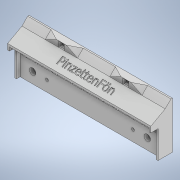
# Autodesk Inventor part: Leitung3-b
Saved by Autodesk Inventor 2020 (Build 240168000, 168)
## iProperties
Created: 2019-09-12
Part Number: Leitung3-b
Material: Generic
Document SubType Name: Modeling
Designer: rainer
Density: 1 g/cm^3
Appearance: Default
Author: rainer
Autodesk Inventor part; units mm, degrees
ref_plane "YZ Plane" through (0, 0, 0) normal (1, 0, 0) x (0, 1, 0)
ref_plane "XZ Plane" through (0, 0, 0) normal (0, 1, 0) x (-1, 0, 0)
sketch "Sketch1" plane through (0, 0, 0) normal (0, 0, 1) x (1, 0, 0)
  line L0 (-100, 17.5) -> (100, 17.5)
  line L1 (100, 17.5) -> (100, -17.5)
  line L2 (100, -17.5) -> (-100, -17.5)
  line L3 (-100, -17.5) -> (-100, 17.5)
  point P0 (0, 0)
  point P1 (0, 17.5)
  point P2 (-100, 0)
  dimension "d0" = 200
  dimension "d1" = 35
  constraints: 8 end point, 2 midpoint, 2 parallel, 1 horizontal, 1 horizontal alignment, 1 perpendicular, 1 vertical alignment
  measures "d0" distance of L0.start L0.end
  measures "d1" distance of L2.end L0.start
extrude "Extrusion1" add sketch "Sketch1" along normal blind 10
ref_plane "Work Plane1" through (0, 0, 30) normal (0, 0, 1) x (1, 0, 0)
sketch "Sketch2" plane through (0, 0, 30) normal (0, 0, 1) x (1, 0, 0)
  line L0 (-100, -17.5) -> (100, -17.5)
  line L1 (100, -17.5) -> (100, 6.5)
  line L2 (100, 6.5) -> (-100, 6.5)
  line L3 (-100, 6.5) -> (-100, -17.5)
  line L4 (100, 17.5) -> (-100, 17.5) projected
  line L5 (-100, -17.5) -> (100, -17.5) projected
  point P0 (0, 0)
  point P1 (0, 6.5)
  dimension "d5" = 24
  dimension "d6" = 200
  dimension "d32" = 0
  constraints: 8 end point, 2 parallel, 1 horizontal, 1 midpoint, 1 perpendicular, 1 vertical alignment
  measures "d5" distance of L2.end L0.start
  measures "d6" distance of L1.end L2.end
  measures "d32" distance between parallel lines of L5 L0
extrude "Extrusion2" add sketch "Sketch2" along normal blind 10
loft "Loft1" add section 1 edges at (0, -17.5, 10) (100, 0, 10) (0, 17.5, 10) (-100, 0, 10) section 2 edges at (0, -17.5, 30) (-100, -5.5, 30) (0, 6.5, 30) (100, -5.5, 30)
sketch "Sketch3" plane through (0, 0, 0) normal (0, 0, -1) x (-1, 0, 0)
  line L0 (-95, 12.5) -> (95, 12.5)
  line L1 (95, 12.5) -> (95, -12.5)
  line L2 (95, -12.5) -> (-95, -12.5)
  line L3 (-95, -12.5) -> (-95, 12.5)
  point P0 (0, 0)
  point P1 (-95, 0)
  point P2 (0, 12.5)
  dimension "d14" = 190
  dimension "d15" = 25
  constraints: 8 end point, 2 midpoint, 2 parallel, 1 horizontal, 1 horizontal alignment, 1 perpendicular, 1 vertical alignment
  measures "d14" distance of L0.start L0.end
  measures "d15" distance of L2.end L0.start
extrude "Extrusion3" cut sketch "Sketch3" against normal blind 10
sketch "Sketch4" plane through (0, 0, 40) normal (0, 0, 1) x (1, 0, 0)
  line L0 (-95, -12.5) -> (95, -12.5)
  line L1 (95, -12.5) -> (95, 3.5)
  line L2 (95, 3.5) -> (-95, 3.5)
  line L3 (-95, 3.5) -> (-95, -12.5)
  line L4 (-100, -17.5) -> (100, -17.5) projected
  point P0 (0, 0)
  point P1 (0, 3.5)
  dimension "d18" = 190
  dimension "d19" = 16
  dimension "d20" = 5
  constraints: 8 end point, 2 parallel, 1 horizontal, 1 midpoint, 1 perpendicular, 1 vertical alignment
  measures "d18" distance of L1.end L2.end
  measures "d19" distance of L2.end L0.start
  measures "d20" distance between parallel lines of L4 L0
extrude "Extrusion4" cut sketch "Sketch4" against normal blind 10
loft "Loft3" cut section 1 edges at (0, 3.5, 30) (-95, -4.5, 30) (0, -12.5, 30) (95, -4.5, 30) section 2 edges at (-95, 0, 10) (0, 12.5, 10) (95, 0, 10) (0, -12.5, 10)
sketch "Sketch6" plane through (0, 0, 40) normal (0, 0, 1) x (1, 0, 0)
  line L0 (-109.7574, -25.248) -> (108.0798, -25.248)
  line L1 (108.0798, -25.248) -> (108.0798, 3.5)
  line L2 (108.0798, 3.5) -> (-109.7574, 3.5)
  line L3 (-109.7574, 3.5) -> (-109.7574, -25.248)
  point P0 (0, 0)
  constraints: 8 end point, 2 parallel, 1 horizontal, 1 perpendicular
extrude "Extrusion6" cut sketch "Sketch6" against normal blind 25
thicken "Thicken2" operation add thickness 10 both sides no extend neighbours yes toward (0, 0, -1) faces at (33.3333, 4.5, 40)
sketch "Sketch7" plane through (-100, -17.5, 0) normal (0, -1, 0) x (1, 0, 0)
  line L0 (200, 0) -> (0, 0) projected
  line L1 (200, 15) -> (0, 15) projected
  line L2 (10, 0) -> (50, 0)
  line L3 (50, 0) -> (50, 15)
  line L4 (50, 15) -> (10, 15)
  line L5 (10, 15) -> (10, 0)
  line L6 (0, 0) -> (0, 15) projected
  line L7 (190, 0) -> (150, 0)
  line L8 (150, 0) -> (150, 15)
  line L9 (150, 15) -> (190, 15)
  line L10 (190, 15) -> (190, 0)
  line L11 (200, 0) -> (200, 15) projected
  point P0 (100, 0)
  point P1 (190, 15)
  point P2 (150, 0)
  point P3 (10, 15)
  dimension "d41" = 40
  dimension "d42" = 10
  dimension "d43" = 40
  dimension "d44" = 10
  constraints: 16 end point, 4 parallel, 4 point on line, 2 horizontal, 2 perpendicular
  measures "d41" distance between parallel lines of L3 L5
  measures "d42" distance between parallel lines of L6 L5
  measures "d43" distance between parallel lines of L10 L8
  measures "d44" distance between parallel lines of L11 L10
extrude "Extrusion7" add sketch "Sketch7" along normal blind 15 contours L0 L8 L1 L10 | L0 L5 L1 L3
sketch "Sketch9" plane through (0, 0, 15) normal (0, 0, 1) x (1, 0, 0)
  line L0 (-90, -17.5) -> (-90, -32.5) projected
  line L1 (-50, -32.5) -> (-90, -32.5) projected
  line L2 (90, -32.5) -> (50, -32.5) projected
  line L3 (50, -17.5) -> (50, -32.5) projected
  line L4 (90, -17.5) -> (90, -32.5) projected
  point P0 (0, 0)
  point P1 (-80, -25)
  point P2 (80, -25)
  dimension "d62" = 10
  dimension "d63" = 7.5
  dimension "d64" = 7.5
  dimension "d73" = 10
  measures "d62" distance from line of L0 point (-80, -25)
  measures "d63" distance from line of L1 point (-80, -25)
  measures "d64" distance from line of L2 point (80, -25)
  measures "d73" distance from line of L4 point (80, -25)
hole "Hole2" at (-80, -25, 15) at (80, -25, 15) direction (0, 0, -1) diameter 4.2 end through all counterbore diameter 9 counterbore depth 5
sketch "Sketch10" plane through (0, 0, 15) normal (0, 0, 1) x (1, 0, 0)
  line L0 (-50, -17.5) -> (-50, -32.5) projected
  line L1 (-50, -32.5) -> (-90, -32.5) projected
  line L2 (50, -17.5) -> (50, -32.5) projected
  point P0 (0, 0)
  point P1 (-60, -25)
  point P2 (60, -25)
  dimension "d74" = 10
  dimension "d75" = 7.5
  dimension "d76" = 10
  measures "d74" distance from line of L0 point (-60, -25)
  measures "d75" distance from line of L1 point (-60, -25)
  measures "d76" distance from line of L2 point (60, -25)
hole "Hole3" at (-60, -25, 15) at (60, -25, 15) direction (0, 0, -1) diameter 4.2 end through all
sketch "Sketch11" plane through (0, 0, 0) normal (0, 0, -1) x (-1, 0, 0)
  line L0 (95, -12.5) -> (-95, -12.5) projected
  line L1 (-95, 12.5) -> (95, 12.5) projected
  line L2 (-75.6667, -12.5) -> (-73.6667, -12.5)
  line L3 (-73.6667, -12.5) -> (-73.6667, 12.5)
  line L4 (-73.6667, 12.5) -> (-75.6667, 12.5)
  line L5 (-75.6667, 12.5) -> (-75.6667, -12.5)
  line L6 (-95, -12.5) -> (-95, 12.5) projected
  point P0 (0, 0)
  dimension "d84" = 2
  dimension "d85" = 19.3333
  constraints: 8 end point, 2 parallel, 2 point on line, 1 horizontal, 1 perpendicular
  measures "d84" distance between parallel lines of L3 L5
  measures "d85" distance between parallel lines of L6 L5
extrude "Extrusion8" add sketch "Sketch11" against normal blind 30 contours L0 L5 L1 L3
pattern_linear "Rectangular Pattern1" count 8 spacing 21.3333 along (-1, 0, 0) of "Extrusion8"
sketch "Sketch12" plane through (100, -17.5, 0) normal (1, 0, 0) x (0, 0, -1)
  line L0 (-30, 21) -> (-30, 24) projected
  line L1 (0, 35) -> (-10, 35) projected
  line L2 (-30, 24) -> (-10, 35)
  line L3 (-10, 35) -> (-34.2959, 35)
  line L4 (-34.2959, 35) -> (-33.7888, 23.828)
  line L5 (-33.7888, 23.828) -> (-30, 24)
  point P0 (0, 17.5)
  constraints: 8 end point, 1 collinear, 1 perpendicular
extrude "Extrusion9" cut sketch "Sketch12" against normal through all
sketch "Sketch13" plane through (100, -17.5, 0) normal (1, 0, 0) x (0, 0, -1)
  line L0 (-31.9216, 3.0257) -> (-15, 3.0257)
  line L1 (-15, 3.0257) -> (-15, 20)
  line L2 (-15, 20) -> (-31.9216, 20)
  line L3 (-31.9216, 20) -> (-31.9216, 3.0257)
  line L4 (-30, 21) -> (-15, 21) projected
  line L5 (-15, 21) -> (-15, 0) projected
  point P0 (0, 17.5)
  dimension "d93" = 1
  dimension "d94" = 0
  constraints: 8 end point, 2 parallel, 1 horizontal, 1 perpendicular
  measures "d93" distance between parallel lines of L4 L2
  measures "d94" distance between parallel lines of L5 L1
extrude "Extrusion10" cut sketch "Sketch13" against normal through all
sketch "Sketch14" plane through (-100, 3.5, 15) normal (0, -1, 0) x (1, 0, 0)
  line L0 (200, 15) -> (0, 15) projected
  line L1 (0, 0) -> (5, 0) projected
  line L2 (0, 15) -> (2.5, 15)
  line L3 (2.5, 15) -> (2.5, 0)
  line L4 (2.5, 0) -> (0, 0)
  line L5 (0, 0) -> (0, 15)
  line L6 (200, -5) -> (200, 15) projected
  line L7 (195, 0) -> (200, 0) projected
  line L8 (200, 15) -> (197.5, 15)
  line L9 (197.5, 15) -> (197.5, 0)
  line L10 (197.5, 0) -> (200, 0)
  line L11 (200, 0) -> (200, 15)
  point P0 (100, -15)
  point P1 (2.5, 15)
  dimension "d97" = 2.5
  dimension "d98" = 2.5
  constraints: 16 end point, 4 parallel, 2 horizontal, 2 midpoint, 2 perpendicular
  measures "d97" distance between parallel lines of L5 L3
  measures "d98" distance between parallel lines of L6 L9
extrude "Extrusion11" add sketch "Sketch14" along normal blind 5
sketch "Sketch15" plane through (0, 0, 15) normal (0, 0, 1) x (1, 0, 0)
  line L0 (-97.5, -1.5) -> (-100, -1.5) projected
  line L1 (-100, -17.5) -> (-97.5, -17.5)
  line L2 (-97.5, -17.5) -> (-97.5, -1.5)
  line L3 (-97.5, -1.5) -> (-100, -1.5)
  line L4 (-100, -1.5) -> (-100, -17.5)
  line L5 (100, -17.5) -> (100, 17.5) projected
  line L6 (97.5, 3.5) -> (97.5, -1.5) projected
  line L7 (100, -17.5) -> (97.5, -17.5)
  line L8 (97.5, -17.5) -> (97.5, -1.5)
  line L9 (97.5, -1.5) -> (100, -1.5)
  line L10 (100, -1.5) -> (100, -17.5)
  line L11 (-97.5, -17.5) -> (-97.5, -15)
  line L12 (97.5, -15) -> (97.5, -17.5)
  point P0 (0, 0)
  constraints: 20 end point, 5 parallel, 2 horizontal, 2 perpendicular, 1 point on line
extrude "Extrusion12" add sketch "Sketch15" along normal blind 5
sketch "Sketch16" plane through (-100, -17.5, 0) normal (-1, 0, 0) x (0, 0, 1)
  line L0 (0, 35) -> (0, 0) projected
  line L1 (0, 35) -> (10, 35)
  line L2 (10, 35) -> (10, 44)
  line L3 (10, 44) -> (0, 44)
  line L4 (0, 44) -> (0, 35)
  line L5 (10, 44) -> (12, 44) construction
  point P0 (0, 17.5)
  dimension "d104" = 10
  dimension "d105" = 9
  constraints: 10 end point, 2 horizontal, 2 parallel, 1 perpendicular
  measures "d104" distance of L3.end L2.end
  measures "d105" distance of L2.end L1.end
extrude "Extrusion13" add sketch "Sketch16" against normal blind 200
sketch "Sketch17" plane through (-100, 17.5, 10) normal (0, 0, 1) x (1, 0, 0)
  line L0 (0, 0) -> (0, 9) projected
  line L1 (200, 0) -> (0, 0) projected
  line L2 (200, 9) -> (200, 0) projected
  point P0 (100, -17.5)
  point P1 (55, 4)
  point P2 (145, 4)
  dimension "d110" = 55
  dimension "d111" = 4
  dimension "d112" = 4
  dimension "d113" = 55
  measures "d110" distance from line of L0 point (55, 4)
  measures "d111" distance from line of L1 point (55, 4)
  measures "d112" distance from line of L1 point (145, 4)
  measures "d113" distance from line of L2 point (145, 4)
hole "Hole4" at (-45, 21.5, 10) at (45, 21.5, 10) direction (0, 0, -1) diameter 4.2 end through all
sketch "Sketch18" plane through (-100, 17.5, 10) normal (0, 0, 1) x (1, 0, 0)
  line L0 (51, 7.5) -> (59, 7.5)
  line L1 (59, 7.5) -> (59, 0.5)
  line L2 (59, 0.5) -> (51, 0.5)
  line L3 (51, 0.5) -> (51, 7.5)
  circle A0 centre (55, 4) radius 2.1 projected
  line L4 (141, 7.5) -> (149, 7.5)
  line L5 (149, 7.5) -> (149, 0.5)
  line L6 (149, 0.5) -> (141, 0.5)
  line L7 (141, 0.5) -> (141, 7.5)
  circle A1 centre (145, 4) radius 2.1 projected
  point P0 (100, -17.5)
  dimension "d121" = 8
  dimension "d122" = 7
  dimension "d123" = 4
  dimension "d124" = 3.5
  dimension "d125" = 8
  dimension "d126" = 7
  dimension "d127" = 3.5
  dimension "d128" = 4
  constraints: 16 end point, 4 parallel, 2 horizontal, 2 perpendicular
  measures "d121" distance of L0.start L0.end
  measures "d122" distance of L2.end L0.start
  measures "d123" distance from line of A0.centre L1
  measures "d124" distance from line of L0 A0.centre
  measures "d125" distance of L4.start L4.end
  measures "d126" distance of L4.end L5.end
  measures "d127" distance from line of A1.centre L4
  measures "d128" distance from line of A1.centre L5
extrude "Extrusion14" cut sketch "Sketch18" along normal blind 5 and the other way blind 5 contours L0 L1 L2 L3 | A0 | L4 L5 L6 L7 | A1
thicken "Thicken3" operation add thickness 22.5 both sides no extend neighbours yes toward (0, -1, 0) faces at (-95.8333, -17.5, 5)
thicken "Thicken4" operation add thickness 22.5 both sides no extend neighbours yes toward (0, -1, 0) faces at (16.6667, -17.5, 10)
thicken "Thicken5" operation add thickness 22.5 both sides no extend neighbours yes toward (0, -1, 0) faces at (95.8333, -17.5, 5)
thicken "Thicken6" operation add thickness 7.5 both sides no extend neighbours yes toward (0, -1, 0) faces at (63.3333, -32.5, 5)
thicken "Thicken7" operation add thickness 7.5 both sides no extend neighbours yes toward (0, -1, 0) faces at (-76.6667, -32.5, 5)
sketch "Sketch20" plane through (-100, 6.5, 30) normal (0, 0.8762159, 0.4819187) x (1, 0, 0)
  line L0 (88.0896, 17.1592) -> (111.9104, 17.1592) construction
  line L1 (111.9104, 17.1592) -> (111.9104, 14.1998) construction
  line L2 (111.9104, 14.1998) -> (88.0896, 14.1998) construction
  line L3 (88.0896, 14.1998) -> (88.0896, 17.1592) construction
  line L4 (200, 22.8254) -> (0, 22.8254) projected
  spline S0 degree 2 poles (68.2577, 14.0717) (68.2577, 13.4234) (67.7958, 12.2564) (67.3825, 11.8512) knots 0 0 0 1 2 2 2
  spline S1 degree 2 poles (67.3825, 11.8512) (66.8639, 11.3407) (65.4619, 10.814) (64.3922, 10.814) knots 0 0 0 1 2 2 2
  line L5 (64.3922, 10.814) -> (63.2658, 10.814)
  line L6 (63.2658, 10.814) -> (63.2658, 7.0862)
  line L7 (63.2658, 7.0862) -> (61.9368, 7.0862)
  line L8 (61.9368, 7.0862) -> (61.9368, 17.0862)
  line L9 (61.9368, 17.0862) -> (64.4489, 17.0862)
  spline S2 degree 2 poles (64.4489, 17.0862) (65.3404, 17.0862) (66.5883, 16.7945) (67.0665, 16.4623) knots 0 0 0 1 2 2 2
  spline S3 degree 2 poles (67.0665, 16.4623) (67.6256, 16.0814) (68.2577, 14.9063) (68.2577, 14.0717) knots 0 0 0 1 2 2 2
  spline S4 degree 2 poles (66.872, 14.0311) (66.872, 14.5498) (66.5154, 15.3115) (66.1507, 15.5546) knots 0 0 0 1 2 2 2
  spline S5 degree 2 poles (66.1507, 15.5546) (65.8347, 15.7653) (64.9919, 15.9355) (64.3679, 15.9355) knots 0 0 0 1 2 2 2
  line L10 (64.3679, 15.9355) -> (63.2658, 15.9355)
  line L11 (63.2658, 15.9355) -> (63.2658, 11.9485)
  line L12 (63.2658, 11.9485) -> (64.1734, 11.9485)
  spline S6 degree 2 poles (64.1734, 11.9485) (64.9838, 11.9485) (65.9806, 12.2078) (66.3047, 12.5482) knots 0 0 0 1 2 2 2
  spline S7 degree 2 poles (66.3047, 12.5482) (66.6045, 12.848) (66.872, 13.553) (66.872, 14.0311) knots 0 0 0 1 2 2 2
  line L13 (70.7131, 7.0862) -> (69.4489, 7.0862)
  line L14 (69.4489, 7.0862) -> (69.4489, 14.5903)
  line L15 (69.4489, 14.5903) -> (70.7131, 14.5903)
  line L16 (70.7131, 14.5903) -> (70.7131, 7.0862)
  line L17 (70.8023, 15.8383) -> (69.3679, 15.8383)
  line L18 (69.3679, 15.8383) -> (69.3679, 17.1511)
  line L19 (69.3679, 17.1511) -> (70.8023, 17.1511)
  line L20 (70.8023, 17.1511) -> (70.8023, 15.8383)
  line L21 (78.4603, 7.0862) -> (77.1961, 7.0862)
  line L22 (77.1961, 7.0862) -> (77.1961, 11.365)
  spline S8 degree 2 poles (77.1961, 11.365) (77.1961, 11.8837) (77.0989, 12.7751) (76.953, 13.0425) knots 0 0 0 1 2 2 2
  spline S9 degree 2 poles (76.953, 13.0425) (76.799, 13.3261) (76.248, 13.6016) (75.778, 13.6016) knots 0 0 0 1 2 2 2
  spline S10 degree 2 poles (75.778, 13.6016) (75.3079, 13.6016) (74.3112, 13.0992) (73.8331, 12.694) knots 0 0 0 1 2 2 2
  line L23 (73.8331, 12.694) -> (73.8331, 7.0862)
  line L24 (73.8331, 7.0862) -> (72.5689, 7.0862)
  line L25 (72.5689, 7.0862) -> (72.5689, 14.5903)
  line L26 (72.5689, 14.5903) -> (73.8331, 14.5903)
  line L27 (73.8331, 14.5903) -> (73.8331, 13.7556)
  spline S11 degree 2 poles (73.8331, 13.7556) (74.4003, 14.2661) (75.4943, 14.801) (76.1102, 14.801) knots 0 0 0 1 2 2 2
  spline S12 degree 2 poles (76.1102, 14.801) (77.2123, 14.801) (78.4603, 13.3423) (78.4603, 11.9566) knots 0 0 0 1 2 2 2
  line L28 (78.4603, 11.9566) -> (78.4603, 7.0862)
  line L29 (85.1621, 7.0862) -> (79.6515, 7.0862)
  line L30 (79.6515, 7.0862) -> (79.6515, 8.0263)
  line L31 (79.6515, 8.0263) -> (83.5737, 13.553)
  line L32 (83.5737, 13.553) -> (79.8136, 13.553)
  line L33 (79.8136, 13.553) -> (79.8136, 14.5903)
  line L34 (79.8136, 14.5903) -> (85.0891, 14.5903)
  line L35 (85.0891, 14.5903) -> (85.0891, 13.6908)
  line L36 (85.0891, 13.6908) -> (81.1507, 8.1478)
  line L37 (81.1507, 8.1478) -> (85.1621, 8.1478)
  line L38 (85.1621, 8.1478) -> (85.1621, 7.0862)
  spline S13 degree 2 poles (89.6029, 6.9161) (87.8039, 6.9161) (85.8266, 8.9339) (85.8266, 10.7978) knots 0 0 0 1 2 2 2
  spline S14 degree 2 poles (85.8266, 10.7978) (85.8266, 12.6292) (87.7472, 14.801) (89.295, 14.801) knots 0 0 0 1 2 2 2
  spline S15 degree 2 poles (89.295, 14.801) (89.9919, 14.801) (91.0697, 14.3958) (91.4668, 13.9663) knots 0 0 0 1 2 2 2
  spline S16 degree 2 poles (91.4668, 13.9663) (91.872, 13.5368) (92.3015, 12.2969) (92.3015, 11.3974) knots 0 0 0 1 2 2 2
  line L39 (92.3015, 11.3974) -> (92.3015, 10.7086)
  line L40 (92.3015, 10.7086) -> (87.107, 10.7086)
  spline S17 degree 2 poles (87.107, 10.7086) (87.107, 9.4039) (88.4198, 8.0182) (89.5867, 8.0182) knots 0 0 0 1 2 2 2
  spline S18 degree 2 poles (89.5867, 8.0182) (90, 8.0182) (90.8023, 8.2046) (91.1264, 8.3504) knots 0 0 0 1 2 2 2
  spline S19 degree 2 poles (91.1264, 8.3504) (91.4668, 8.5125) (91.9368, 8.7961) (92.0908, 8.9258) knots 0 0 0 1 2 2 2
  line L41 (92.0908, 8.9258) -> (92.1637, 8.9258)
  line L42 (92.1637, 8.9258) -> (92.1637, 7.5482)
  spline S20 degree 2 poles (92.1637, 7.5482) (91.9449, 7.459) (91.2804, 7.1997) (91.0211, 7.1268) knots 0 0 0 1 2 2 2
  spline S21 degree 2 poles (91.0211, 7.1268) (90.6564, 7.0214) (90.0567, 6.9161) (89.6029, 6.9161) knots 0 0 0 1 2 2 2
  spline S22 degree 2 poles (91.0697, 11.673) (91.0535, 12.1835) (90.8428, 12.929) (90.6402, 13.1802) knots 0 0 0 1 2 2 2
  spline S23 degree 2 poles (90.6402, 13.1802) (90.4214, 13.4639) (89.7326, 13.7637) (89.222, 13.7637) knots 0 0 0 1 2 2 2
  spline S24 degree 2 poles (89.222, 13.7637) (88.7196, 13.7637) (88.0146, 13.4639) (87.7229, 13.1721) knots 0 0 0 1 2 2 2
  spline S25 degree 2 poles (87.7229, 13.1721) (87.4392, 12.8723) (87.1475, 12.1511) (87.107, 11.673) knots 0 0 0 1 2 2 2
  line L43 (87.107, 11.673) -> (91.0697, 11.673)
  spline S26 degree 2 poles (95.8509, 6.9404) (94.8217, 6.9404) (93.6629, 8.1154) (93.6629, 9.3877) knots 0 0 0 1 2 2 2
  line L44 (93.6629, 9.3877) -> (93.6629, 13.5449)
  line L45 (93.6629, 13.5449) -> (92.812, 13.5449)
  line L46 (92.812, 13.5449) -> (92.812, 14.5903)
  line L47 (92.812, 14.5903) -> (93.6629, 14.5903)
  line L48 (93.6629, 14.5903) -> (93.6629, 16.7459)
  line L49 (93.6629, 16.7459) -> (94.9271, 16.7459)
  line L50 (94.9271, 16.7459) -> (94.9271, 14.5903)
  line L51 (94.9271, 14.5903) -> (97.2528, 14.5903)
  line L52 (97.2528, 14.5903) -> (97.2528, 13.5449)
  line L53 (97.2528, 13.5449) -> (94.9271, 13.5449)
  line L54 (94.9271, 13.5449) -> (94.9271, 9.9712)
  spline S27 degree 2 poles (94.9271, 9.9712) (94.9271, 9.4039) (94.9676, 8.7799) (95.1054, 8.5125) knots 0 0 0 1 2 2 2
  spline S28 degree 2 poles (95.1054, 8.5125) (95.2188, 8.2775) (95.7293, 8.0425) (96.1669, 8.0425) knots 0 0 0 1 2 2 2
  spline S29 degree 2 poles (96.1669, 8.0425) (96.4749, 8.0425) (97.0502, 8.2289) (97.1799, 8.2856) knots 0 0 0 1 2 2 2
  line L55 (97.1799, 8.2856) -> (97.2528, 8.2856)
  line L56 (97.2528, 8.2856) -> (97.2528, 7.1511)
  spline S30 degree 2 poles (97.2528, 7.1511) (96.8963, 7.0538) (96.1669, 6.9404) (95.8509, 6.9404) knots 0 0 0 1 2 2 2
  spline S31 degree 2 poles (100.4538, 6.9404) (99.4246, 6.9404) (98.2658, 8.1154) (98.2658, 9.3877) knots 0 0 0 1 2 2 2
  line L57 (98.2658, 9.3877) -> (98.2658, 13.5449)
  line L58 (98.2658, 13.5449) -> (97.4149, 13.5449)
  line L59 (97.4149, 13.5449) -> (97.4149, 14.5903)
  line L60 (97.4149, 14.5903) -> (98.2658, 14.5903)
  line L61 (98.2658, 14.5903) -> (98.2658, 16.7459)
  line L62 (98.2658, 16.7459) -> (99.53, 16.7459)
  line L63 (99.53, 16.7459) -> (99.53, 14.5903)
  line L64 (99.53, 14.5903) -> (101.8558, 14.5903)
  line L65 (101.8558, 14.5903) -> (101.8558, 13.5449)
  line L66 (101.8558, 13.5449) -> (99.53, 13.5449)
  line L67 (99.53, 13.5449) -> (99.53, 9.9712)
  spline S32 degree 2 poles (99.53, 9.9712) (99.53, 9.4039) (99.5705, 8.7799) (99.7083, 8.5125) knots 0 0 0 1 2 2 2
  spline S33 degree 2 poles (99.7083, 8.5125) (99.8217, 8.2775) (100.3323, 8.0425) (100.7699, 8.0425) knots 0 0 0 1 2 2 2
  spline S34 degree 2 poles (100.7699, 8.0425) (101.0778, 8.0425) (101.6532, 8.2289) (101.7828, 8.2856) knots 0 0 0 1 2 2 2
  line L68 (101.7828, 8.2856) -> (101.8558, 8.2856)
  line L69 (101.8558, 8.2856) -> (101.8558, 7.1511)
  spline S35 degree 2 poles (101.8558, 7.1511) (101.4992, 7.0538) (100.7699, 6.9404) (100.4538, 6.9404) knots 0 0 0 1 2 2 2
  spline S36 degree 2 poles (106.0454, 6.9161) (104.2464, 6.9161) (102.269, 8.9339) (102.269, 10.7978) knots 0 0 0 1 2 2 2
  spline S37 degree 2 poles (102.269, 10.7978) (102.269, 12.6292) (104.1896, 14.801) (105.7374, 14.801) knots 0 0 0 1 2 2 2
  spline S38 degree 2 poles (105.7374, 14.801) (106.4344, 14.801) (107.5122, 14.3958) (107.9092, 13.9663) knots 0 0 0 1 2 2 2
  spline S39 degree 2 poles (107.9092, 13.9663) (108.3144, 13.5368) (108.7439, 12.2969) (108.7439, 11.3974) knots 0 0 0 1 2 2 2
  line L70 (108.7439, 11.3974) -> (108.7439, 10.7086)
  line L71 (108.7439, 10.7086) -> (103.5494, 10.7086)
  spline S40 degree 2 poles (103.5494, 10.7086) (103.5494, 9.4039) (104.8622, 8.0182) (106.0292, 8.0182) knots 0 0 0 1 2 2 2
  spline S41 degree 2 poles (106.0292, 8.0182) (106.4425, 8.0182) (107.2447, 8.2046) (107.5689, 8.3504) knots 0 0 0 1 2 2 2
  spline S42 degree 2 poles (107.5689, 8.3504) (107.9092, 8.5125) (108.3793, 8.7961) (108.5332, 8.9258) knots 0 0 0 1 2 2 2
  line L72 (108.5332, 8.9258) -> (108.6062, 8.9258)
  line L73 (108.6062, 8.9258) -> (108.6062, 7.5482)
  spline S43 degree 2 poles (108.6062, 7.5482) (108.3874, 7.459) (107.7229, 7.1997) (107.4635, 7.1268) knots 0 0 0 1 2 2 2
  spline S44 degree 2 poles (107.4635, 7.1268) (107.0989, 7.0214) (106.4992, 6.9161) (106.0454, 6.9161) knots 0 0 0 1 2 2 2
  spline S45 degree 2 poles (107.5122, 11.673) (107.4959, 12.1835) (107.2853, 12.929) (107.0827, 13.1802) knots 0 0 0 1 2 2 2
  spline S46 degree 2 poles (107.0827, 13.1802) (106.8639, 13.4639) (106.175, 13.7637) (105.6645, 13.7637) knots 0 0 0 1 2 2 2
  spline S47 degree 2 poles (105.6645, 13.7637) (105.1621, 13.7637) (104.4571, 13.4639) (104.1653, 13.1721) knots 0 0 0 1 2 2 2
  spline S48 degree 2 poles (104.1653, 13.1721) (103.8817, 12.8723) (103.59, 12.1511) (103.5494, 11.673) knots 0 0 0 1 2 2 2
  line L74 (103.5494, 11.673) -> (107.5122, 11.673)
  line L75 (115.9157, 7.0862) -> (114.6515, 7.0862)
  line L76 (114.6515, 7.0862) -> (114.6515, 11.365)
  spline S49 degree 2 poles (114.6515, 11.365) (114.6515, 11.8837) (114.5543, 12.7751) (114.4084, 13.0425) knots 0 0 0 1 2 2 2
  spline S50 degree 2 poles (114.4084, 13.0425) (114.2545, 13.3261) (113.7034, 13.6016) (113.2334, 13.6016) knots 0 0 0 1 2 2 2
  spline S51 degree 2 poles (113.2334, 13.6016) (112.7634, 13.6016) (111.7666, 13.0992) (111.2885, 12.694) knots 0 0 0 1 2 2 2
  line L77 (111.2885, 12.694) -> (111.2885, 7.0862)
  line L78 (111.2885, 7.0862) -> (110.0243, 7.0862)
  line L79 (110.0243, 7.0862) -> (110.0243, 14.5903)
  line L80 (110.0243, 14.5903) -> (111.2885, 14.5903)
  line L81 (111.2885, 14.5903) -> (111.2885, 13.7556)
  spline S52 degree 2 poles (111.2885, 13.7556) (111.8558, 14.2661) (112.9498, 14.801) (113.5656, 14.801) knots 0 0 0 1 2 2 2
  spline S53 degree 2 poles (113.5656, 14.801) (114.6677, 14.801) (115.9157, 13.3423) (115.9157, 11.9566) knots 0 0 0 1 2 2 2
  line L82 (115.9157, 11.9566) -> (115.9157, 7.0862)
  line L83 (123.7682, 15.9031) -> (119.1167, 15.9031)
  line L84 (119.1167, 15.9031) -> (119.1167, 13.083)
  line L85 (119.1167, 13.083) -> (123.5737, 13.083)
  line L86 (123.5737, 13.083) -> (123.5737, 11.8999)
  line L87 (123.5737, 11.8999) -> (119.1167, 11.8999)
  line L88 (119.1167, 11.8999) -> (119.1167, 7.0862)
  line L89 (119.1167, 7.0862) -> (117.7877, 7.0862)
  line L90 (117.7877, 7.0862) -> (117.7877, 17.0862)
  line L91 (117.7877, 17.0862) -> (123.7682, 17.0862)
  line L92 (123.7682, 17.0862) -> (123.7682, 15.9031)
  spline S54 degree 2 poles (131.0292, 10.8383) (131.0292, 8.942) (129.2058, 6.8755) (127.6823, 6.8755) knots 0 0 0 1 2 2 2
  spline S55 degree 2 poles (127.6823, 6.8755) (126.1183, 6.8755) (124.3274, 9.0068) (124.3274, 10.8383) knots 0 0 0 1 2 2 2
  spline S56 degree 2 poles (124.3274, 10.8383) (124.3274, 12.7183) (126.175, 14.801) (127.6823, 14.801) knots 0 0 0 1 2 2 2
  spline S57 degree 2 poles (127.6823, 14.801) (129.2058, 14.801) (131.0292, 12.7264) (131.0292, 10.8383) knots 0 0 0 1 2 2 2
  spline S58 degree 2 poles (129.7245, 10.8383) (129.7245, 12.2969) (128.6629, 13.7151) (127.6823, 13.7151) knots 0 0 0 1 2 2 2
  spline S59 degree 2 poles (127.6823, 13.7151) (126.7018, 13.7151) (125.6321, 12.2969) (125.6321, 10.8383) knots 0 0 0 1 2 2 2
  spline S60 degree 2 poles (125.6321, 10.8383) (125.6321, 9.4201) (126.7018, 7.9614) (127.6823, 7.9614) knots 0 0 0 1 2 2 2
  spline S61 degree 2 poles (127.6823, 7.9614) (128.6548, 7.9614) (129.7245, 9.3958) (129.7245, 10.8383) knots 0 0 0 1 2 2 2
  line L93 (126.9773, 15.8464) -> (125.624, 15.8464)
  line L94 (125.624, 15.8464) -> (125.624, 17.1592)
  line L95 (125.624, 17.1592) -> (126.9773, 17.1592)
  line L96 (126.9773, 17.1592) -> (126.9773, 15.8464)
  line L97 (129.7488, 15.8464) -> (128.3955, 15.8464)
  line L98 (128.3955, 15.8464) -> (128.3955, 17.1592)
  line L99 (128.3955, 17.1592) -> (129.7488, 17.1592)
  line L100 (129.7488, 17.1592) -> (129.7488, 15.8464)
  line L101 (138.2172, 7.0862) -> (136.953, 7.0862)
  line L102 (136.953, 7.0862) -> (136.953, 11.365)
  spline S62 degree 2 poles (136.953, 11.365) (136.953, 11.8837) (136.8558, 12.7751) (136.7099, 13.0425) knots 0 0 0 1 2 2 2
  spline S63 degree 2 poles (136.7099, 13.0425) (136.5559, 13.3261) (136.0049, 13.6016) (135.5348, 13.6016) knots 0 0 0 1 2 2 2
  spline S64 degree 2 poles (135.5348, 13.6016) (135.0648, 13.6016) (134.0681, 13.0992) (133.59, 12.694) knots 0 0 0 1 2 2 2
  line L103 (133.59, 12.694) -> (133.59, 7.0862)
  line L104 (133.59, 7.0862) -> (132.3258, 7.0862)
  line L105 (132.3258, 7.0862) -> (132.3258, 14.5903)
  line L106 (132.3258, 14.5903) -> (133.59, 14.5903)
  line L107 (133.59, 14.5903) -> (133.59, 13.7556)
  spline S65 degree 2 poles (133.59, 13.7556) (134.1572, 14.2661) (135.2512, 14.801) (135.8671, 14.801) knots 0 0 0 1 2 2 2
  spline S66 degree 2 poles (135.8671, 14.801) (136.9692, 14.801) (138.2172, 13.3423) (138.2172, 11.9566) knots 0 0 0 1 2 2 2
  line L108 (138.2172, 11.9566) -> (138.2172, 7.0862)
  point P0 (100, 23.154)
  point P1 (100, 17.1592)
  point P2 (100, 22.8254)
  point P3 (141, 22.8254)
  point P4 (59, 22.8254)
  constraints: 2 midpoint, 1 vertical alignment, 2 other
emboss "Emboss1" sketch "Sketch20" operation cut depth 0.5 direction (0, -0.8762159, -0.4819187)
sketch "Sketch21" plane through (100, -1.5, 30) normal (1, 0, 0) x (0, 0, -1)
  line L0 (20, 19) -> (29.0868, 28.0868)
  line L1 (20, 19) -> (32.8506, 19) construction
  line L2 (29.0868, 28.0868) -> (29, 28)
  line L3 (20, 28) -> (30, 28) projected
  line L4 (29, 28) -> (20, 28)
  line L5 (20, 19) -> (0, 8) projected
  line L6 (20, 28) -> (20, 19)
  point P0 (30, 1.5)
  dimension "d145" = 45
  constraints: 10 end point, 2 horizontal, 2 point on line, 1 equal length, 1 perpendicular
  measures "d145" angle of L1 L0
extrude "Extrusion15" cut sketch "Sketch21" against normal blind 50
sketch "Sketch22" plane through (-100, -1.5, 30) normal (-1, 0, 0) x (0, 0, 1)
  line L0 (-20, 19) -> (-29.0717, 28.0717)
  line L1 (-20, 19) -> (-7.1707, 19) construction
  line L2 (-20, 28) -> (-30, 28) projected
  line L3 (-29, 28) -> (-20, 28)
  line L4 (-20, 28) -> (-20, 19)
  point P0 (-30, 1.5)
  dimension "d148" = 135
  constraints: 8 end point, 2 point on line, 1 collinear, 1 equal length, 1 horizontal
  measures "d148" angle of L1 L0
extrude "Extrusion16" cut sketch "Sketch22" against normal blind 50
ref_plane "Work Plane2" through (-40, 18, 10) normal (-1, 0, 0) x (0, 0, 1)
sketch "Sketch23" plane through (-40, 18, 10) normal (-1, 0, 0) x (0, 0, 1)
  line L0 (0, -0.5) -> (0, 8.5) projected
  line L1 (0, 8.5) -> (-9, 8.5) projected
  line L2 (0, -0.5) -> (-9, 8.5)
  line L3 (-9, 8.5) -> (0, 8.5)
  line L4 (0, 8.5) -> (0, -0.5)
  point P0 (-10, -18)
  constraints: 6 end point, 1 collinear, 1 perpendicular
extrude "Extrusion17" cut sketch "Sketch23" against normal blind 80
chamfer "Chamfer1" distance 17.48 angle 20 1 edges at (-50, 22, 5.5) measured on face at (-50.5, 22, 5.5)
chamfer "Chamfer3" distance 1.37 angle 20 1 edges at (-45, 18, 10) measured on face at (-45, 18, 9.5)
chamfer "Chamfer4" distance 1.37 angle 20 1 edges at (45, 18, 10) measured on face at (45, 18, 9.5)
chamfer "Chamfer5" distance 17.48 angle 20 1 edges at (-40, 22, 5.5) measured on face at (-39.5, 22, 5.5)
chamfer "Chamfer6" distance 17.48 angle 20 1 edges at (50, 22, 5.5) measured on face at (50.5, 22, 5.5)
chamfer "Chamfer7" distance 17.48 angle 20 1 edges at (40, 22, 5.5) measured on face at (39.5, 22, 5.5)
thicken "Thicken8" operation add thickness 1 both sides no extend neighbours yes toward (0, -1, 0) faces at (-46.6667, 26.5, 3.9992)
body "Solid1"
